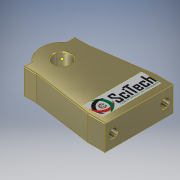
# Autodesk Inventor part: bearing
Saved by Autodesk Inventor 2017 (Build 210142000, 142)
## iProperties
Created: 2019-12-31
Part Number: bearing
Material: Gold
Document SubType Name: Modeling
Designer: Admin
Density: 19.3 g/cm^3
Appearance: Gold - Metal
Mass: 133.588 g
Surface Area: 29.005 cm^2
Volume: 6.92164 cm^3
Author: Admin
Autodesk Inventor part; units mm, degrees
ref_plane "YZ Plane" through (0, 0, 0) normal (1, 0, 0) x (0, 1, 0)
ref_plane "XZ Plane" through (0, 0, 0) normal (0, 1, 0) x (-1, 0, 0)
ref_plane "XY Plane" through (0, 0, 0) normal (0, 0, 1) x (1, 0, 0)
sketch "Sketch1" plane through (0, 0, 0) normal (0, 1, 0) x (-1, 0, 0)
  circle A0 centre (0, 0) radius 3.175
  arc A1 (4.7625, -6.35) -> (4.7625, 6.35) centre (0, 0) ccw
  line L0 (-28.575, 12.7) -> (-28.575, -12.7)
  line L1 (-28.575, -12.7) -> (-22.225, -12.7)
  line L2 (-28.575, 12.7) -> (-22.225, 12.7)
  line L3 (4.7625, -9.525) -> (0, -9.525)
  line L4 (4.7625, 9.525) -> (0, 9.525)
  line L5 (0, -9.525) -> (-22.225, -12.7)
  line L6 (0, 9.525) -> (-22.225, 12.7)
  line L7 (4.7625, 9.525) -> (4.7625, 6.35)
  line L8 (4.7625, -6.35) -> (4.7625, -9.525)
  point P0 (-28.575, 0)
  point P1 (4.7625, 0)
  dimension "d0" = 6.35
  dimension "d1" = 15.875
  dimension "d2" = 25.4
  dimension "d3" = 19.05
  dimension "d5" = 6.35
  dimension "d6" = 6.35
  dimension "d7" = 4.7625
  dimension "d8" = 4.7625
  dimension "d9" = 28.575
  dimension "d12" = 98.13
  dimension "d13" = 98.13
  dimension "d14" = 0
  dimension "d15" = 0
  constraints: 18 end point, 4 horizontal, 3 vertical, 2 centre point, 2 coincident, 2 horizontal alignment, 2 point on circle, 1 midpoint
  measures "d0" diameter of A0
  measures "d1" diameter of A1
  measures "d2" distance of L0.start L0.end
  measures "d3" distance of L4.start L3.start
  measures "d5" distance of L0.start L2.end
  measures "d6" distance of L0.end L1.end
  measures "d7" distance of L4.start L4.end
  measures "d8" distance of L3.start L3.end
  measures "d9" distance from line of point (0, 0) L0
  measures "d12" angle of L6 L7
  measures "d13" angle of L7 L5
  measures "d14" distance between parallel lines of L7 L8
  measures "d15" distance from line of point (4.763, 0) L7
extrude "Extrusion1" add sketch "Sketch1" along normal blind 9.525
sketch "Sketch2" plane through (28.575, 0, 12.7) normal (1, 0, 0) x (0, 0, -1)
  line L0 (0, 0) -> (25.4, 0) projected
  line L1 (25.4, 0) -> (25.4, 9.525) projected
  line L2 (0, 9.525) -> (25.4, 9.525) projected
  line L3 (0, 0) -> (0, 9.525) projected
  circle A0 centre (3.175, 4.7625) radius 1.6654
  circle A1 centre (22.225, 4.7625) radius 1.6717
  point P0 (12.7, 0)
  dimension "d16" = 19.05
  dimension "d17" = 9.525
  constraints: 2 centre point
  measures "d16" distance of A0.centre A1.centre
  measures "d17" horizontal distance of A1.centre point (12.7, 0)
hole "Hole1" at (28.575, 4.7625, 9.525) at (28.575, 4.7625, -9.525) direction (-1, 0, 0) diameter 2.54 depth 9.906 tip angle 118 counterbore diameter 3.175 counterbore depth 7.112
fillet "Fillet1" radius 0.3175 32 edges at (28.575, 0, 0) (25.4, 0, 12.7) (11.1125, 0, 11.1125) (-2.3813, 0, 9.525) (-4.7625, 0, 7.9375) (-7.9375, 0, 0) (-4.7625, 0, -7.9375) (-2.3813, 0, -9.525) (11.1125, 0, -11.1125) (25.4, 0, -12.7) (28.575, 9.525, 0) (25.4, 9.525, -12.7) (11.1125, 9.525, -11.1125) (-2.3813, 9.525, -9.525) (-4.7625, 9.525, -7.9375) (-7.9375, 9.525, 0) (-4.7625, 9.525, 7.9375) (-2.3813, 9.525, 9.525) (11.1125, 9.525, 11.1125) (25.4, 9.525, 12.7) (22.225, 4.7625, 12.7) (0, 4.7625, 9.525) (-4.7625, 4.7625, 9.525) (-4.7625, 4.7625, 6.35) (0, 4.7625, -9.525) (22.225, 4.7625, -12.7) (-4.7625, 4.7625, -9.525) (-4.7625, 4.7625, -6.35) (3.175, 0, 0) (3.175, 9.525, 0) (28.575, 4.7625, -12.7) (28.575, 4.7625, 12.7)
fillet "Fillet2" radius 0.3175 2 edges at (28.575, 4.7625, -7.9375) (28.575, 4.7625, 11.1125)
sketch "Sketch3" plane through (0, 9.525, 0) normal (0, 1, 0) x (1, 0, 0)
  line L0 (18.7817, -11.0314) -> (18.7817, 10.6001) construction
  line L1 (18.7817, 10.6001) -> (26.0293, 10.6001) construction
  line L2 (26.0293, 10.6001) -> (26.0293, -11.0314) construction
  line L3 (26.0293, -11.0314) -> (18.7817, -11.0314) construction
  point P0 (0, 0)
  constraints: 2 other
equation "\"d8\" = d7"
body "Solid1"
